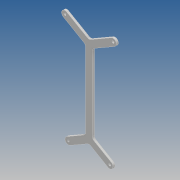
# Autodesk Inventor part: Tall Handle
Saved by Autodesk Inventor 2017 (Build 210142000, 142)
## iProperties
Created: 2017-07-19
Part Number: Tall Handle
Material: Generic
Document SubType Name: Modeling
Designer: yella
Density: 1 g/cm^3
Appearance: Default
Author: yella
Autodesk Inventor part; units mm, degrees
ref_plane "YZ Plane" through (0, 0, 0) normal (1, 0, 0) x (0, 1, 0)
ref_plane "XZ Plane" through (0, 0, 0) normal (0, 1, 0) x (-1, 0, 0)
ref_plane "XY Plane" through (0, 0, 0) normal (0, 0, 1) x (1, 0, 0)
sketch "Sketch1" plane through (0, 0, 0) normal (0, 1, 0) x (-1, 0, 0)
  circle A0 centre (-30.6147, -73.9104) radius 1.6
  circle A1 centre (-30.6147, -73.9104) radius 1.6
  circle A2 centre (-30.6147, -73.9104) radius 1.6
  circle A3 centre (-30.6147, -73.9104) radius 1.6
  circle A4 centre (-35.5945, 85.9327) radius 1.6
  circle A5 centre (35.5991, 85.9437) radius 1.6
  circle A6 centre (30.6147, -73.9104) radius 1.6
  line L0 (0, 0) -> (5, 0)
  line L1 (0, 0) -> (-5, 0)
  line L2 (35.5991, 85.9437) -> (70.9318, 85.9437) construction
  arc A7 (38.0991, 81.6136) -> (33.0991, 90.2738) centre (35.5991, 85.9437) ccw
  line L3 (33.0991, 90.2738) -> (5, 74.0508)
  line L4 (38.0991, 81.6136) -> (7.5, 63.9472)
  arc A8 (-33.0991, 90.2738) -> (-38.0991, 81.6136) centre (-35.5991, 85.9437) ccw
  line L5 (-33.0991, 90.2738) -> (-5, 74.0508)
  line L6 (-38.0991, 81.6136) -> (-7.5, 63.9472)
  line L7 (5, 74.0508) -> (2.5, 72.6075)
  line L8 (-5, 74.0508) -> (-2.5, 72.6075)
  line L9 (30.6147, -73.9104) -> (60.192, -73.9104) construction
  line L10 (-30.6147, -73.9104) -> (-1.0374, -73.9104) construction
  arc A9 (28.1147, -78.2405) -> (33.1147, -69.5802) centre (30.6147, -73.9104) ccw
  line L11 (30.6147, -73.9104) -> (28.1147, -78.2405) construction
  line L12 (30.6147, -73.9104) -> (35.6147, -73.9104) construction
  line L13 (33.1147, -69.5802) -> (7.5, -54.7916)
  line L14 (28.1147, -78.2405) -> (5, -64.8952)
  arc A10 (-33.0991, -69.6073) -> (-28.1303, -78.2134) centre (-30.6147, -73.9104) ccw
  line L15 (-28.1303, -78.2134) -> (-5, -64.8952)
  line L16 (-33.0991, -69.6073) -> (-7.5051, -54.8705)
  line L17 (5, -64.8952) -> (2.5034, -63.4538)
  line L18 (-2.4915, -63.4509) -> (-5, -64.8952)
  line L19 (5, 59.6171) -> (5, -50.4615)
  line L20 (-5, -50.5375) -> (-5, 59.6171)
  arc A11 (7.5, 63.9472) -> (5, 59.6171) centre (10, 59.6171) ccw
  arc A12 (5, -50.4615) -> (7.5, -54.7916) centre (10, -50.4615) ccw
  arc A13 (2.5034, -63.4538) -> (-2.4915, -63.4509) centre (0.0034, -67.7839) ccw
  arc A14 (-7.5051, -54.8705) -> (-5, -50.5375) centre (-10, -50.5375) ccw
  arc A15 (-2.5, 72.6075) -> (2.5, 72.6075) centre (0, 76.9376) ccw
  arc A16 (-5, 59.6171) -> (-7.5, 63.9472) centre (-10, 59.6171) ccw
  point P0 (0.0068, -62.0124)
  dimension "d0" = 5
  dimension "d1" = 5
  dimension "d3" = 5
  dimension "d6" = 5
  dimension "d7" = 120
  dimension "d8" = 5
  constraints: 42 end point, 20 point on circle, 17 centre point, 12 tangent, 6 horizontal, 5 coincident, 5 equal radius, 3 parallel, 3 point on line, 1 equal length, 1 vertical
  measures "d0" distance of L0.start L0.end
  measures "d1" distance of L0.start L1.end
  measures "d3" radius of A7
  measures "d6" radius of A9
  measures "d7" angle of L11 L12
  measures "d8" radius of A11
extrude "Extrusion1" add sketch "Sketch1" along normal blind 3
body "Solid1"
